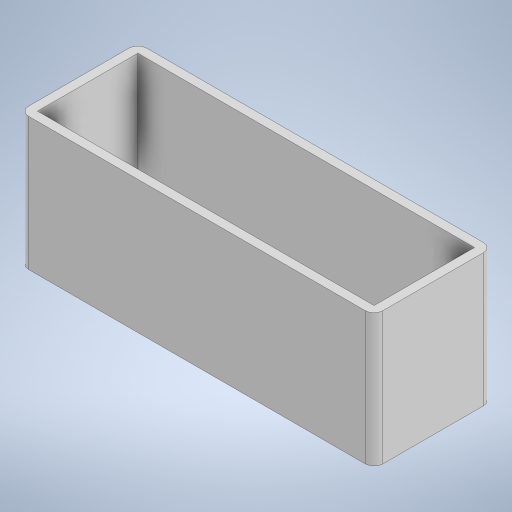
# Autodesk Inventor part: beetkasten
Saved by Autodesk Inventor 2023 (Build 270158000, 158)
## iProperties
Created: 2025-06-13
Part Number: beetkasten
Material: Generisch
Document SubType Name: Modeling
Designer: johan
Density: 1 g/cm^3
Appearance: Vorgabe
Author: johan
Autodesk Inventor part; units mm, degrees
ref_plane "YZ Plane" through (0, 0, 0) normal (1, 0, 0) x (0, 1, 0)
ref_plane "XZ Plane" through (0, 0, 0) normal (0, 1, 0) x (-1, 0, 0)
ref_plane "XY Plane" through (0, 0, 0) normal (0, 0, 1) x (1, 0, 0)
sketch "Skizze1" plane through (0, 0, 0) normal (0, 0, 1) x (1, 0, 0)
  line L0 (-300, 0.252) -> (300, 0.252)
  line L1 (300, 0.252) -> (300, 250.252)
  line L2 (300, 250.252) -> (-300, 250.252)
  line L3 (-300, 250.252) -> (-300, 0.252)
  point P0 (0, 0)
  dimension "d0" = 600
  dimension "d1" = 250
  constraints: 8 end point, 2 parallel, 1 horizontal, 1 perpendicular
  measures "d0" distance of L2.end L1.end
  measures "d1" distance of L1.end L0.end
extrude "Extrusion1" add sketch "Skizze1" along normal mid plane 200
sketch "Skizze2" plane through (-300, 250.252, 100) normal (0, 1, 0) x (1, 0, 0)
  line L0 (600, 0) -> (0, 0) projected
  line L1 (600, 200) -> (600, 0) projected
  line L2 (15, 0) -> (585, 0)
  line L3 (600, 15) -> (600, 185)
  line L4 (585, 200) -> (15, 200)
  line L5 (0, 185) -> (0, 15)
  arc A0 (0, 15) -> (15, 0) centre (15, 15) ccw
  arc A1 (15, 200) -> (0, 185) centre (15, 185) ccw
  arc A2 (600, 185) -> (585, 200) centre (585, 185) ccw
  arc A3 (585, 0) -> (600, 15) centre (585, 15) ccw
  line L6 (0, 200) -> (0, 0) projected
  line L7 (0, 200) -> (600, 200) projected
  line L8 (0, 0) -> (600, 0)
  line L9 (600, 0) -> (600, 200)
  line L10 (600, 200) -> (0, 200)
  line L11 (0, 200) -> (0, 0)
  point P0 (300, 100)
  point P1 (585, 0)
  dimension "d4" = 15
  constraints: 16 end point, 8 point on circle, 8 tangent, 4 centre point, 4 parallel, 4 point on line, 3 equal radius, 2 horizontal, 2 perpendicular
  measures "d4" radius of A0
extrude "Extrusion2" cut sketch "Skizze2" against normal through all contours L0 A3 L1 | L0 L6 A0 | A2 L7 L1 | L6 L7 A1
sketch "Skizze3" plane through (-285, 250.252, 100) normal (0, 1, 0) x (1, 0, 0)
  arc A0 (0, 200) -> (-15, 185) centre (0, 185) ccw projected
  arc A1 (570, 0) -> (585, 15) centre (570, 15) ccw projected
  line L0 (0, 185) -> (570, 185)
  line L1 (570, 185) -> (570, 15)
  line L2 (570, 15) -> (0, 15)
  line L3 (0, 15) -> (0, 185)
  point P0 (285, 100)
  constraints: 8 end point, 2 parallel, 1 horizontal, 1 perpendicular
extrude "Extrusion3" cut sketch "Skizze3" against normal blind 235
sketch "Skizze4" plane through (0, 0, 0) normal (1, 0, 0) x (0, 1, 0)
  line L0 (225, 85) -> (225, -110.1417)
  line L1 (250.252, -85) -> (15.252, -85) projected
  line L2 (225, 85) -> (225, 112.4289)
  line L3 (225, 112.4289) -> (265.8438, 112.4289)
  line L4 (265.8438, 112.4289) -> (265.8438, -110.1417)
  line L5 (265.8438, -110.1417) -> (225, -110.1417)
  point P0 (0, 0)
  constraints: 10 end point, 2 perpendicular, 1 horizontal, 1 vertical
extrude "Extrusion4" cut sketch "Skizze4" along normal through all both and the other way through all
